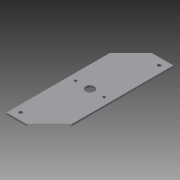
# Autodesk Inventor part: motor support plate
Saved by Autodesk Inventor 2015 SP1 (Build 190203100, 203)
## iProperties
Created: 2015-01-27
Part Number: motor support plate
Material: Generic
Document SubType Name: Modeling
Designer: Admin
Density: 1 g/cm^3
Appearance: Default
Author: Admin
Autodesk Inventor part; units mm, degrees
ref_plane "YZ Plane" through (0, 0, 0) normal (1, 0, 0) x (0, 1, 0)
ref_plane "XZ Plane" through (0, 0, 0) normal (0, 1, 0) x (-1, 0, 0)
ref_plane "XY Plane" through (0, 0, 0) normal (0, 0, 1) x (1, 0, 0)
sketch "Sketch1" plane through (0, 0, 0) normal (0, 1, 0) x (-1, 0, 0)
  line L0 (0, 0) -> (-76.2, 0)
  line L1 (-76.2, 0) -> (-76.2, -222.25)
  line L2 (-76.2, -222.25) -> (0, -222.25)
  line L3 (0, -222.25) -> (0, 0)
  dimension "d0" = 76.2
  dimension "d1" = 222.25
  constraints: 8 end point, 2 parallel, 1 horizontal, 1 perpendicular
  measures "d0" distance of L2.end L1.end
  measures "d1" distance of L1.end L0.end
extrude "Extrusion1" add sketch "Sketch1" along normal blind 3.175
sketch "Sketch2" plane through (0, 3.175, 0) normal (0, 1, 0) x (1, 0, 0)
  line L0 (0, 0) -> (76.2, 0) projected
  line L1 (0, 222.25) -> (0, 0) projected
  circle A0 centre (12.7, 111.125) radius 2.54
  circle A1 centre (63.5, 111.125) radius 2.54
  circle A2 centre (38.1, 111.125) radius 7.9375
  dimension "d4" = 111.125
  dimension "d5" = 38.1
  dimension "d6" = 25.4
  dimension "d7" = 25.4
  dimension "d8" = 111.125
  dimension "d9" = 111.125
  dimension "d10" = 5.08
  dimension "d11" = 5.08
  dimension "d12" = 15.875
  constraints: 3 centre point, 3 coincident
  measures "d4" distance from line of L0 point (38.1, 111.125)
  measures "d5" distance from line of L1 point (38.1, 111.125)
  measures "d6" distance of point (12.7, 111.125) point (38.1, 111.125)
  measures "d7" distance of point (63.5, 111.125) point (38.1, 111.125)
  measures "d8" distance from line of L0 point (12.7, 111.125)
  measures "d9" distance from line of L0 point (63.5, 111.125)
  measures "d10" diameter of A0
  measures "d11" diameter of A1
  measures "d12" diameter of A2
extrude "Extrusion2" cut sketch "Sketch2" against normal blind 25.4
sketch "Sketch3" plane through (0, 3.175, 0) normal (0, 1, 0) x (1, 0, 0)
  line L0 (0, 0) -> (76.2, 0) projected
  line L1 (76.2, 0) -> (76.2, 222.25) projected
  line L2 (76.2, 222.25) -> (0, 222.25) projected
  line L3 (0, 222.25) -> (0, 0) projected
  point P0 (12.7, 12.7)
  point P1 (63.5, 12.7)
  point P2 (63.5, 209.55)
  point P3 (12.7, 209.55)
  dimension "d15" = 12.7
  dimension "d16" = 12.7
  dimension "d17" = 12.7
  dimension "d18" = 12.7
  dimension "d19" = 12.7
  dimension "d20" = 12.7
  dimension "d21" = 12.7
  dimension "d22" = 12.7
  measures "d15" distance from line of L0 point (12.7, 12.7)
  measures "d16" distance from line of L3 point (12.7, 12.7)
  measures "d17" distance from line of L0 point (63.5, 12.7)
  measures "d18" distance from line of L1 point (63.5, 12.7)
  measures "d19" distance from line of L3 point (12.7, 209.55)
  measures "d20" distance from line of L2 point (12.7, 209.55)
  measures "d21" distance from line of L2 point (63.5, 209.55)
  measures "d22" distance from line of L1 point (63.5, 209.55)
hole "Hole1" at (12.7, 3.175, -12.7) at (63.5, 3.175, -12.7) at (63.5, 3.175, -209.55) at (12.7, 3.175, -209.55) direction (0, -1, 0) diameter 6.35 end through all
body "Solid1"
